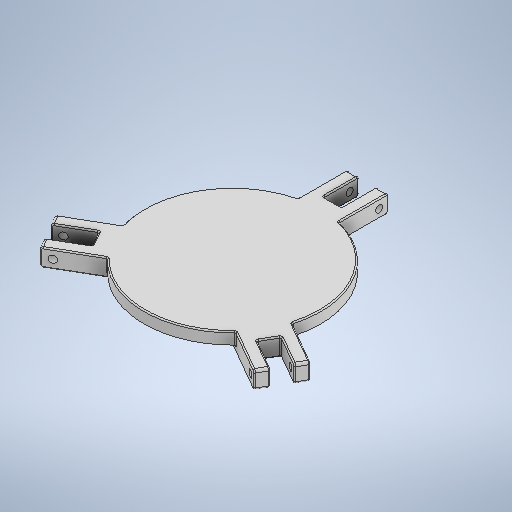
# Autodesk Inventor part: Base Móvel II
Saved by Autodesk Inventor 2025.3 (Build 293356000, 356)
## iProperties
Created: 2025-03-23
Part Number: Base Móvel II
Material: Generic
Document SubType Name: Modeling
Designer: erikg
Density: 1 g/cm^3
Appearance: Default
Author: erikg
Autodesk Inventor part; units mm, degrees
note: some values were not read from the file. Chosen so that the rebuilt part matches the saved one: direction of "Hole1".
ref_plane "YZ Plane" through (0, 0, 0) normal (1, 0, 0) x (0, 1, 0)
ref_plane "XZ Plane" through (0, 0, 0) normal (0, 1, 0) x (-1, 0, 0)
ref_plane "XY Plane" through (0, 0, 0) normal (0, 0, 1) x (1, 0, 0)
sketch "Sketch1" plane through (0, 0, 0) normal (0, 1, 0) x (-1, 0, 0)
  circle A0 centre (0, 0) radius 75
  dimension "d0" = 150
  constraints: 1 centre point, 1 coincident
  measures "d0" diameter of A0
extrude "Extrusion1" add sketch "Sketch1" along normal blind 10
sketch "Sketch2" plane through (0, 10, 0) normal (0, 1, 0) x (1, 0, 0)
  line L0 (-17.5, 65) -> (17.5, 65)
  line L1 (17.5, 65) -> (17.5, 115)
  line L2 (17.5, 115) -> (-17.5, 115)
  line L3 (-17.5, 115) -> (-17.5, 65)
  circle A0 centre (0, 0) radius 75 projected
  line L4 (-7.5, 115) -> (7.5, 115)
  line L5 (7.5, 115) -> (7.5, 85)
  line L6 (7.5, 85) -> (-7.5, 85)
  line L7 (-7.5, 85) -> (-7.5, 115)
  line L8 (-47.5417, -47.6554) -> (-65.0417, -17.3446)
  line L9 (-65.0417, -17.3446) -> (-108.3429, -42.3446)
  line L10 (-108.3429, -42.3446) -> (-90.8429, -72.6554)
  line L11 (-90.8429, -72.6554) -> (-47.5417, -47.6554)
  line L12 (-95.8429, -63.9952) -> (-103.3429, -51.0048)
  line L13 (-103.3429, -51.0048) -> (-77.3622, -36.0048)
  line L14 (-77.3622, -36.0048) -> (-69.8622, -48.9952)
  line L15 (-69.8622, -48.9952) -> (-95.8429, -63.9952)
  line L16 (65.0417, -17.3446) -> (47.5417, -47.6554)
  line L17 (47.5417, -47.6554) -> (90.8429, -72.6554)
  line L18 (90.8429, -72.6554) -> (108.3429, -42.3446)
  line L19 (108.3429, -42.3446) -> (65.0417, -17.3446)
  line L20 (103.3429, -51.0048) -> (95.8429, -63.9952)
  line L21 (95.8429, -63.9952) -> (69.8622, -48.9952)
  line L22 (69.8622, -48.9952) -> (77.3622, -36.0048)
  line L23 (77.3622, -36.0048) -> (103.3429, -51.0048)
  point P0 (0, 65)
  point P1 (0, 85)
  point P2 (-17.5, 72.9298)
  point P3 (17.5, 72.9298)
  point P4 (-56.2917, -32.5)
  point P5 (-73.6122, -42.5)
  point P6 (56.2917, -32.5)
  point P7 (73.6122, -42.5)
  point P8 (71.909, -21.3094)
  point P9 (54.409, -51.6203)
  point P10 (-54.409, -51.6203)
  point P11 (-71.909, -21.3094)
  dimension "d3" = 65
  dimension "d4" = 50
  dimension "d5" = 35
  dimension "d6" = 30
  dimension "d7" = 15
  dimension "d12" = 360
  constraints: 48 end point, 4 parallel, 3 point on line, 2 horizontal, 2 midpoint, 2 perpendicular, 2 vertical alignment, 55 other
  measures "d3" vertical distance of A0.centre L0.start
  measures "d4" distance of L2.end L0.start
  measures "d5" distance of L1.end L2.end
  measures "d6" distance of L6.end L4.start
  measures "d7" distance of L5.end L6.end
extrude "Extrusion2" add sketch "Sketch2" against normal blind 15 contours L3 A0 L1 L0 | L3 L2 L7 L6 L5 L1 A0 | L9 L8 L11 A0 | A0 L11 L10 L15 L14 L13 L9 | L19 L18 L23 L22 L21 L17 A0 | A0 L17 L16 L19
sketch "Sketch3" plane through (108.3429, -5, 42.3446) normal (0.5, 0, -0.8660254) x (-0.8660254, 0, -0.5)
  line L0 (0, 15) -> (0, 0) projected
  point P0 (115, 5)
  point P1 (8, 7.5)
  point P2 (0, 7.5)
  dimension "d14" = 8
  constraints: 1 midpoint
  measures "d14" distance of point (0, 7.5) point (8, 7.5)
hole "Hole1" at (101.4147, 2.5, 38.3446) direction (-0.5, 0, 0.8660254) diameter 6 depth 35
sketch "Sketch4" plane through (17.5, 10, -72.9298) normal (1, 0, 0) x (0, 0, -1)
  line L0 (42.0702, 0) -> (42.0702, -15) projected
  line L1 (12.0702, 0) -> (12.0702, -15) projected
  point P0 (-72.9298, -10)
  point P1 (34.0702, -7.5)
  point P2 (42.0702, -7.5)
  dimension "d22" = 8
  dimension "d23" = 22
  constraints: 1 midpoint
  measures "d22" distance of point (42.07, -7.5) point (34.07, -7.5)
  measures "d23" distance from line of L1 point (34.07, -7.5)
hole "Hole2" at (17.5, 2.5, -107) direction (-1, 0, 0) diameter 6 end through all
sketch "Sketch5" plane through (-108.3429, -5, 42.3446) normal (-0.5, 0, -0.8660254) x (-0.8660254, 0, 0.5)
  line L0 (0, 15) -> (0, 0) projected
  point P0 (-115, 5)
  point P1 (-8, 7.5)
  dimension "d31" = 8
  measures "d31" distance from line of L0 point (-8, 7.5)
hole "Hole3" at (-101.4147, 2.5, 38.3446) direction (0.5, 0, 0.8660254) diameter 6 end through all
fillet "Fillet1" radius 2 12 edges at (93.3429, 10, 68.3253) (93.3429, -5, 68.3253) (105.8429, -5, 46.6747) (105.8429, 10, 46.6747) (12.5, 10, -115) (12.5, -5, -115) (-12.5, -5, -115) (-93.3429, 10, 68.3253) (-93.3429, -5, 68.3253) (-105.8429, 10, 46.6747) (-105.8429, -5, 46.6747) (-12.5, 10, -115)
fillet "Fillet2" radius 1 22 edges at (0, -5, -65) (0, 0, -65) (17.5, 0, -68.9649) (-17.5, 0, -68.9649) (17.5, -2.5, -65) (-17.5, -2.5, -65) (17.5, 5, -72.9298) (-17.5, 5, -72.9298) (-71.909, 5, 21.3094) (-68.4753, 0, 19.327) (-65.0417, -2.5, 17.3446) (-56.2917, 0, 32.5) (-50.9753, 0, 49.6379) (-47.5417, -2.5, 47.6554) (-54.409, 5, 51.6203) (71.909, 5, 21.3094) (68.4753, 0, 19.327) (65.0417, -2.5, 17.3446) (54.409, 5, 51.6203) (47.5417, -2.5, 47.6554) (56.2917, 0, 32.5) (50.9753, 0, 49.6379)
fillet "Fillet3" radius 1 6 edges at (-7.5, 2.5, -85) (7.5, 2.5, -85) (69.8622, 2.5, 48.9952) (77.3622, 2.5, 36.0048) (-77.3622, 2.5, 36.0048) (-69.8622, 2.5, 48.9952)
fillet "Fillet4" radius 1 95 edges at (17.2071, -4.7071, -65.2929) (17.5, -4.4142, -114.4142) (17.5, 2.5, -115) (17.5, 9.4142, -114.4142) (17.5, 10, -93.357) (17.7115, 10, -73.0989) (64.9519, 10, -37.5) (72.1613, 10, 21.2108) (89.5995, 10, 31.523) (107.8356, 9.4142, 42.0517) (108.3429, 2.5, 42.3446) (107.8356, -4.4142, 42.0517) (86.2593, -5, 29.5946) (65.1489, -5, 17.7447) (56.2917, -5, 32.5) (47.9418, -5, 47.5482) (68.7593, -5, 59.9054) (90.3356, -4.4142, 72.3626) (90.8429, 2.5, 72.6554) (90.3356, 9.4142, 72.3626) (72.0995, 10, 61.8339) (54.4498, 10, 51.8881) (0, 10, 75) (-54.4498, 10, 51.8881) (-72.0995, 10, 61.8339) (-90.3356, 9.4142, 72.3626) (-90.8429, 2.5, 72.6554) (-90.3356, -4.4142, 72.3626) (-68.7593, -5, 59.9054) (-47.9418, -5, 47.5482) (-56.2917, -5, 32.5) (-65.1489, -5, 17.7447) (-86.2593, -5, 29.5946) (-107.8356, -4.4142, 42.0517) (-108.3429, 2.5, 42.3446) (-107.8356, 9.4142, 42.0517) (-89.5995, 10, 31.523) (-72.1613, 10, 21.2108) (-64.9519, 10, -37.5) (-17.7115, 10, -73.0989) (-17.5, 10, -93.357) (-17.5, 9.4142, -114.4142) (-17.5, 2.5, -115) (-17.5, -4.4142, -114.4142) (-17.5, -5, -89.5) (-17.2071, -4.7071, -65.2929) (17.5, -5, -89.5) (-7.2071, -5, -85.2929) (0, -5, -85) (7.2071, -5, -85.2929) (7.5, -5, -99.5) (7.5, -4.4142, -114.4142) (7.5, 2.5, -115) (7.5, 9.4142, -114.4142) (7.5, 10, -99.5) (7.2071, 10, -85.2929) (0, 10, -85) (-7.2071, 10, -85.2929) (-7.5, 10, -99.5) (-7.5, 9.4142, -114.4142) (-7.5, 2.5, -115) (-7.5, -4.4142, -114.4142) (-7.5, -5, -99.5) (70.2623, -5, 48.888) (82.4195, -5, 56.2452) (95.3356, -4.4142, 63.7023) (95.8429, 2.5, 63.9952) (95.3356, 9.4142, 63.7023) (82.4195, 10, 56.2452) (70.2623, 10, 48.888) (73.6122, 10, 42.5) (77.4694, 10, 36.4049) (89.9195, 10, 43.2548) (102.8356, 9.4142, 50.7119) (103.3429, 2.5, 51.0048) (102.8356, -4.4142, 50.7119) (89.9195, -5, 43.2548) (77.4694, -5, 36.4049) (73.6122, -5, 42.5) (-102.8356, -4.4142, 50.7119) (-103.3429, 2.5, 51.0048) (-102.8356, 9.4142, 50.7119) (-89.9195, 10, 43.2548) (-77.4694, 10, 36.4049) (-73.6122, 10, 42.5) (-70.2623, 10, 48.888) (-82.4195, 10, 56.2452) (-95.3356, 9.4142, 63.7023) (-95.8429, 2.5, 63.9952) (-95.3356, -4.4142, 63.7023) (-82.4195, -5, 56.2452) (-70.2623, -5, 48.888) (-73.6122, -5, 42.5) (-77.4694, -5, 36.4049) (-89.9195, -5, 43.2548)
body "Solid1"
